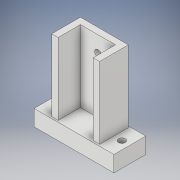
# Autodesk Inventor part: XPulleySupportBase
Saved by Autodesk Inventor 2019 (Build 230136000, 136)
## iProperties
Created: 2019-08-19
Part Number: XPulleySupportBase
Material: ABS Plastic
Document SubType Name: Modeling
Designer: Bruno
Density: 1.06 g/cm^3
Appearance: Smooth - White
Author: Bruno
## iProperties of the stored document XPulleySupportBase_3DPrint.ipt
Created: 2019-09-09
Part Number: XPulleySupportBase_3DPrint
Material: Generic
Document SubType Name: Modeling
Designer: Bruno
Density: 1 g/cm^3
Appearance: Default
Author: Bruno
Autodesk Inventor part; units mm, degrees
ref_plane "YZ Plane" through (0, 0, 0) normal (1, 0, 0) x (0, 1, 0)
ref_plane "XZ Plane" through (0, 0, 0) normal (0, 1, 0) x (-1, 0, 0)
ref_plane "XY Plane" through (0, 0, 0) normal (0, 0, 1) x (1, 0, 0)
sketch "Sketch2" plane through (0, 0, 0) normal (0, 1, 0) x (-1, 0, 0)
  line L0 (10.6557, -7.541) -> (-39.3443, -7.541)
  line L1 (-39.3443, -7.541) -> (-39.3443, 12.459)
  line L2 (-39.3443, 12.459) -> (10.6557, 12.459)
  line L3 (10.6557, 12.459) -> (10.6557, -7.541)
  point P0 (0, 0)
  dimension "d10" = 20
  dimension "d11" = 50
  constraints: 8 end point, 2 parallel, 1 horizontal, 1 perpendicular
  measures "d10" distance of L2.end L0.start
  measures "d11" distance of L0.start L0.end
extrude "Extrusion3" add sketch "Sketch2" along normal blind 10
sketch "Sketch3" plane through (0, 10, 0) normal (0, 1, 0) x (1, 0, 0)
  line L0 (39.3443, 7.541) -> (-10.6557, 7.541) projected
  line L1 (-10.6557, 7.541) -> (-10.6557, -12.459) projected
  line L2 (-10.6557, -12.459) -> (39.3443, -12.459) projected
  line L3 (39.3443, -12.459) -> (39.3443, 7.541) projected
  line L4 (-0.6557, -11.459) -> (-0.6557, 6.541)
  line L5 (-0.6557, 6.541) -> (29.3443, 6.541)
  line L6 (29.3443, 6.541) -> (29.3443, -11.459)
  line L7 (29.3443, -11.459) -> (25.3443, -11.459)
  line L8 (25.3443, -11.459) -> (25.3443, 2.541)
  line L9 (25.3443, 2.541) -> (3.3443, 2.541)
  line L10 (3.3443, 2.541) -> (3.3443, -11.459)
  line L11 (3.3443, -11.459) -> (-0.6557, -11.459)
  line L12 (-0.6557, 6.541) -> (-10.6557, 6.541) construction
  line L13 (29.3443, 6.541) -> (39.3443, 6.541) construction
  line L14 (-0.6557, 6.541) -> (-0.6557, 7.541) construction
  point P0 (0, 0)
  dimension "d14" = 22
  dimension "d15" = 4
  dimension "d16" = 4
  dimension "d17" = 1
  dimension "d18" = 14
  constraints: 22 end point, 9 perpendicular, 5 point on line, 2 collinear, 1 vertical
  measures "d14" distance of L8.end L9.end
  measures "d15" distance of L6.end L7.end
  measures "d16" distance between parallel lines of L5 L9
  measures "d17" distance of L4.end L14.end
  measures "d18" distance of L9.end L10.end
extrude "Extrusion4" add sketch "Sketch3" along normal blind 45 contours L4 L5 L6 L7 L8 L9 L10 L11
sketch "Sketch4" plane through (29.3443, 10, -6.541) normal (0, 0, -1) x (-1, 0, 0)
  circle A0 centre (15, 34.875) radius 2.125
  line L0 (15, 34.875) -> (0, 34.875) construction
  line L1 (0, 0) -> (0, 45) projected
  line L2 (15, 34.875) -> (30, 34.875) construction
  line L3 (30, 0) -> (30, 45) projected
  line L4 (0, 45) -> (30, 45) projected
  point P0 (29.3443, -10)
  point P1 (28, 0)
  dimension "d21" = 4.25
  dimension "d22" = 8
  constraints: 4 end point, 2 point on line, 1 centre point, 1 collinear, 1 horizontal, 2 other
  measures "d21" diameter of A0
  measures "d22" distance edge to line of A0 L4
extrude "Extrusion5" cut sketch "Sketch4" against normal up to next
sketch "Sketch5" plane through (0, 10, 0) normal (0, 1, 0) x (1, 0, 0)
  circle A0 centre (-5.6557, -2.459) radius 2.125
  circle A1 centre (34.3443, -2.459) radius 2.125
  line L0 (-5.6557, -2.459) -> (-10.6557, -2.459) construction
  line L1 (34.3443, -2.459) -> (39.3443, -2.459) construction
  line L2 (39.3443, -12.459) -> (39.3443, 7.541) projected
  line L3 (39.3443, 7.541) -> (-10.6557, 7.541) projected
  line L4 (-10.6557, 7.541) -> (-10.6557, -12.459) projected
  point P0 (0, 0)
  dimension "d26" = 4.25
  dimension "d27" = 10
  dimension "d28" = 5
  constraints: 4 end point, 2 centre point, 2 collinear, 2 horizontal, 2 midpoint, 1 equal radius
  measures "d26" diameter of A0
  measures "d27" distance between parallel lines of L3 L0
  measures "d28" distance of L0.start L0.end
extrude "Extrusion6" cut sketch "Sketch5" against normal up to next
body "Solid2"
